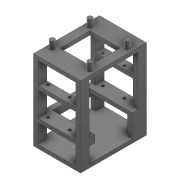
# Autodesk Inventor part: support
Saved by Autodesk Inventor 2021 (Build 250183000, 183)
## iProperties
Created: 2021-02-15
Part Number: support
Material: Generic
Document SubType Name: Modeling
Designer: lobato
Density: 1 g/cm^3
Appearance: Default
Author: lobato
Autodesk Inventor part; units mm, degrees
ref_plane "YZ Plane" through (0, 0, 0) normal (1, 0, 0) x (0, 1, 0)
ref_plane "XZ Plane" through (0, 0, 0) normal (0, 1, 0) x (-1, 0, 0)
sketch "Sketch1" plane through (0, 0, 0) normal (0, 1, 0) x (-1, 0, 0)
  line L0 (25, 35) -> (-25, 35)
  line L1 (-25, 35) -> (-25, -35)
  line L2 (-25, -35) -> (25, -35)
  line L3 (25, -35) -> (25, 35)
  line L4 (25, 35) -> (-25, -35) construction
  line L5 (-25, 35) -> (25, -35) construction
  point P0 (0, 0)
  dimension "d0" = 50
  dimension "d1" = 70
  constraints: 12 end point, 2 midpoint, 2 parallel, 1 horizontal, 1 perpendicular
  measures "d0" distance of L2.end L1.end
  measures "d1" distance of L1.end L0.end
extrude "Extrusion1" add sketch "Sketch1" along normal blind 4
sketch "Sketch2" plane through (0, 4, 0) normal (0, 1, 0) x (1, 0, 0)
  line L0 (25, -35) -> (25, 35) projected
  line L1 (25, 35) -> (-25, 35) projected
  line L2 (25, -35) -> (20, -35)
  line L3 (20, -35) -> (20, 35)
  line L4 (20, 35) -> (25, 35)
  line L5 (25, 35) -> (25, -35)
  line L6 (-25, 35) -> (-25, -35) projected
  line L7 (-25, -35) -> (-20, -35)
  line L8 (-20, -35) -> (-20, 35)
  line L9 (-20, 35) -> (-25, 35)
  line L10 (-25, 35) -> (-25, -35)
  point P0 (0, 0)
  dimension "d4" = 5
  dimension "d5" = 5
  dimension "d6" = 70
  constraints: 16 end point, 4 parallel, 2 horizontal, 2 perpendicular, 1 point on line
  measures "d4" distance of L3.end L4.end
  measures "d5" distance of L9.end L8.end
  measures "d6" distance of L8.end L7.end
extrude "Extrusion2" add sketch "Sketch2" along normal blind 20
sketch "Sketch3" plane through (0, 24, 0) normal (0, 1, 0) x (1, 0, 0)
  line L0 (-25, -35) -> (25, -35) projected
  line L1 (25, -35) -> (25, 35) projected
  line L2 (-25, -35) -> (25, -35)
  line L3 (25, -35) -> (25, 35)
  line L4 (25, 35) -> (-25, 35)
  line L5 (-25, 35) -> (-25, -35)
  line L6 (-20, -20) -> (20, -20)
  line L7 (20, -20) -> (20, 20)
  line L8 (20, 20) -> (-20, 20)
  line L9 (-20, 20) -> (-20, -20)
  line L10 (-20, -20) -> (20, 20) construction
  line L11 (20, -20) -> (-20, 20) construction
  line L12 (-15.5, -29) -> (7.5, -29) construction
  line L13 (7.5, -29) -> (7.5, 29) construction
  line L14 (7.5, 29) -> (-15.5, 29) construction
  line L15 (-15.5, 29) -> (-15.5, -29) construction
  circle A0 centre (-15.5, -29) radius 1.5
  circle A1 centre (-15.5, 29) radius 1.5
  circle A2 centre (7.5, 29) radius 1.5
  circle A3 centre (7.5, -29) radius 1.5
  point P0 (0, 0)
  dimension "d9" = 40
  dimension "d10" = 40
  dimension "d13" = 23
  dimension "d14" = 58
  dimension "d15" = 6
  dimension "d16" = 4.5
  dimension "d17" = 3
  dimension "d18" = 3
  dimension "d19" = 3
  dimension "d20" = 3
  constraints: 28 end point, 6 parallel, 4 centre point, 4 coincident, 3 horizontal, 3 perpendicular, 2 midpoint
  measures "d9" distance of L8.end L7.end
  measures "d10" distance of L7.end L6.end
  measures "d13" distance of L14.end L13.end
  measures "d14" distance of L13.end L12.end
  measures "d15" distance between parallel lines of L0 L12
  measures "d16" distance between parallel lines of L9 L15
  measures "d17" diameter of A0
  measures "d18" diameter of A1
  measures "d19" diameter of A2
  measures "d20" diameter of A3
extrude "Extrusion3" add sketch "Sketch3" along normal blind 4
sketch "Sketch4" plane through (-25, 0, -35) normal (-1, 0, 0) x (0, 0, 1)
  line L0 (9, 20) -> (61, 20)
  line L1 (61, 20) -> (61, 4)
  line L2 (61, 4) -> (9, 4)
  line L3 (9, 4) -> (9, 20)
  line L4 (0, 28) -> (70, 28) projected
  line L5 (0, 0) -> (0, 28) projected
  point P0 (35, 0)
  dimension "d21" = 52
  dimension "d22" = 16
  dimension "d23" = 8
  dimension "d24" = 9
  constraints: 8 end point, 2 parallel, 1 horizontal, 1 perpendicular
  measures "d21" distance of L1.end L2.end
  measures "d22" distance of L0.end L1.end
  measures "d23" distance between parallel lines of L0 L4
  measures "d24" distance between parallel lines of L5 L3
extrude "Extrusion4" cut sketch "Sketch4" against normal blind 5
sketch "Sketch5" plane through (0, 28, 0) normal (0, 1, 0) x (1, 0, 0)
  line L0 (25, 35) -> (-25, 35) projected
  line L1 (-20, 35) -> (-20, 26) projected
  line L2 (-25, 35) -> (-20, 35)
  line L3 (-20, 35) -> (-20, 26)
  line L4 (-20, 26) -> (-25, 26)
  line L5 (-25, 26) -> (-25, 35)
  line L6 (-25, -35) -> (25, -35) projected
  line L7 (20, -20) -> (20, -35) projected
  line L8 (25, -35) -> (20, -35)
  line L9 (20, -35) -> (20, -26)
  line L10 (20, -26) -> (25, -26)
  line L11 (25, -26) -> (25, -35)
  line L12 (-25, 35) -> (-25, -35) projected
  line L13 (-20, -26) -> (-20, -35) projected
  line L14 (-25, -35) -> (-20, -35)
  line L15 (-20, -35) -> (-20, -26)
  line L16 (-20, -26) -> (-25, -26)
  line L17 (-25, -26) -> (-25, -35)
  line L18 (20, -35) -> (20, 35) projected
  line L19 (25, 35) -> (20, 35)
  line L20 (20, 35) -> (20, 26)
  line L21 (20, 26) -> (25, 26)
  line L22 (25, 26) -> (25, 35)
  point P0 (0, 0)
  dimension "d27" = 9
  dimension "d28" = 9
  constraints: 32 end point, 8 parallel, 4 horizontal, 4 perpendicular, 2 point on line
  measures "d27" distance of L2.end L1.end
  measures "d28" distance of L8.end L9.end
extrude "Extrusion5" add sketch "Sketch5" along normal blind 53 contours L22 L21 L18 L0 | L1 L4 L5 L0 | L10 L11 L6 L7 | L16 L13 L6 L12
sketch "Sketch6" plane through (0, 81, 0) normal (0, 1, 0) x (1, 0, 0)
  line L0 (-25, 35) -> (-25, -35) projected
  line L1 (20, -35) -> (25, -35) projected
  line L2 (-25, 35) -> (25, 35)
  line L3 (25, 35) -> (25, -35)
  line L4 (25, -35) -> (-25, -35)
  line L5 (-25, -35) -> (-25, 35)
  line L6 (-10, -10) -> (10, -10) construction
  line L7 (10, -10) -> (10, 10) construction
  line L8 (10, 10) -> (-10, 10) construction
  line L9 (-10, 10) -> (-10, -10) construction
  line L10 (-10, -10) -> (10, 10) construction
  line L11 (10, -10) -> (-10, 10) construction
  line L12 (-25, 25) -> (25, 25) construction
  line L13 (25, 25) -> (25, -25) construction
  line L14 (25, -25) -> (-25, -25) construction
  line L15 (-25, -25) -> (-25, 25) construction
  line L16 (-25, 25) -> (25, -25) construction
  line L17 (25, 25) -> (-25, -25) construction
  line L18 (20, 20) -> (20, -20) construction
  line L19 (-20, 20) -> (20, 20) construction
  line L20 (20, 20) -> (20, -20) construction
  line L21 (20, -20) -> (-20, -20) construction
  line L22 (-20, -20) -> (-20, 20) construction
  line L23 (-20, 20) -> (20, -20) construction
  line L24 (20, 20) -> (-20, -20) construction
  line L25 (-16, 16) -> (16, 16)
  line L26 (16, 16) -> (16, -16)
  line L27 (16, -16) -> (-16, -16)
  line L28 (-16, -16) -> (-16, 16)
  line L29 (-16, 16) -> (16, -16) construction
  line L30 (16, 16) -> (-16, -16) construction
  point P0 (0, 0)
  dimension "d31" = 20
  dimension "d32" = 20
  dimension "d33" = 50
  dimension "d34" = 50
  dimension "d35" = 40
  dimension "d36" = 40
  dimension "d37" = 32
  dimension "d38" = 32
  constraints: 56 end point, 10 parallel, 8 midpoint, 5 horizontal, 5 perpendicular
  measures "d31" distance of L8.end L7.end
  measures "d32" distance of L7.end L6.end
  measures "d33" distance of L13.end L14.end
  measures "d34" distance of L12.end L13.end
  measures "d35" distance of L18.end L21.end
  measures "d36" distance of L19.end L18.end
  measures "d37" distance of L26.end L27.end
  measures "d38" distance of L25.end L26.end
extrude "Extrusion6" add sketch "Sketch6" along normal blind 4
sketch "Sketch7" plane through (0, 85, 0) normal (0, 1, 0) x (1, 0, 0)
  line L0 (20, 20) -> (20, -20) construction
  line L1 (-20, 20) -> (20, 20) construction
  line L2 (20, 20) -> (20, -20) construction
  line L3 (20, -20) -> (-20, -20) construction
  line L4 (-20, -20) -> (-20, 20) construction
  line L5 (-20, 20) -> (20, -20) construction
  line L6 (20, 20) -> (-20, -20) construction
  circle A0 centre (-20, 20) radius 2.5
  line L7 (-20, 20) -> (20, 20) projected
  circle A1 centre (20, 20) radius 2.5
  circle A2 centre (20, -20) radius 2.5
  line L8 (20, -20) -> (-20, -20) projected
  circle A3 centre (-20, -20) radius 2.5
  point P0 (0, 0)
  dimension "d41" = 40
  dimension "d42" = 40
  dimension "d43" = 5
  dimension "d44" = 5
  dimension "d45" = 5
  dimension "d46" = 5
  constraints: 12 end point, 4 centre point, 4 coincident, 2 midpoint, 2 parallel, 1 horizontal, 1 perpendicular
  measures "d41" distance of L0.end L3.end
  measures "d42" distance of L1.end L0.end
  measures "d43" diameter of A0
  measures "d44" diameter of A1
  measures "d45" diameter of A2
  measures "d46" diameter of A3
extrude "Extrusion7" add sketch "Sketch7" along normal blind 8
sketch "Sketch8" plane through (25, 0, 35) normal (1, 0, 0) x (0, 0, -1)
  line L0 (15, 28) -> (55, 28) projected
  line L1 (9, 4) -> (61, 4) projected
  line L2 (15, 28) -> (55, 28)
  line L3 (55, 28) -> (55, 4)
  line L4 (55, 4) -> (15, 4)
  line L5 (15, 4) -> (15, 28)
  point P0 (15, 4)
  dimension "d53" = 40
  constraints: 8 end point, 2 parallel, 1 horizontal, 1 perpendicular, 1 point on line
  measures "d53" distance of L3.end L4.end
extrude "Extrusion8" cut sketch "Sketch8" against normal blind 5
ref_plane "Work Plane1" through (0, 58, 0) normal (0, 1, 0) x (1, 0, 0)
sketch "Sketch9" plane through (0, 58, 0) normal (0, 1, 0) x (1, 0, 0)
  line L0 (-20, -26) -> (-20, -35) projected
  line L1 (20, -35) -> (20, -26) projected
  line L2 (-20, -35) -> (20, -35)
  line L3 (20, -35) -> (20, -26)
  line L4 (20, -26) -> (-20, -26)
  line L5 (-20, -26) -> (-20, -35)
  line L6 (-25, 26) -> (-20, 26) projected
  line L7 (25, 35) -> (-25, 35) projected
  line L8 (-20, 26) -> (20, 26)
  line L9 (20, 26) -> (20, 35)
  line L10 (20, 35) -> (-20, 35)
  line L11 (-20, 35) -> (-20, 26)
  circle A0 centre (-15.5, -29) radius 1.5 projected
  circle A1 centre (-15.5, -29) radius 1.25
  circle A2 centre (7.5, -29) radius 1.5 projected
  circle A3 centre (7.5, -29) radius 1.25
  circle A4 centre (-15.5, 29) radius 1.5 projected
  circle A5 centre (-15.5, 29) radius 1.25
  circle A6 centre (7.5, 29) radius 1.5 projected
  circle A7 centre (7.5, 29) radius 1.25
  point P0 (0, 0)
  point P1 (-20, 35)
  constraints: 16 end point, 4 centre point, 4 coincident, 4 parallel, 2 horizontal, 2 perpendicular, 2 point on line
extrude "Extrusion9" add sketch "Sketch9" against normal blind 4 contours L4 L1 L2 L0 | L9 L8 L11 L7
sketch "Sketch10" plane through (25, 0, 35) normal (1, 0, 0) x (0, 0, -1)
  line L0 (61, 20) -> (9, 20) projected
  line L1 (15, 4) -> (15, 28) projected
  line L2 (9, 20) -> (15, 20)
  line L3 (15, 20) -> (15, 4)
  line L4 (15, 4) -> (9, 4)
  line L5 (9, 4) -> (9, 20)
  point P0 (35, 0)
  point P1 (15, 20)
  constraints: 8 end point, 2 parallel, 1 horizontal, 1 perpendicular
extrude "Extrusion10" cut sketch "Sketch10" against normal blind 5
body "Solid1"
